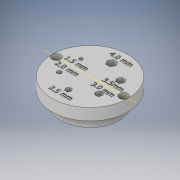
# Autodesk Inventor part: AllenKeyHolder
Saved by Autodesk Inventor 2019.1 (Build 231200000, 200)
## iProperties
Created: 2018-08-31
Part Number: AllenKeyHolder
Material: Generic
Document SubType Name: Modeling
Designer: steele
Density: 1 g/cm^3
Appearance: Default
Author: steele
Autodesk Inventor part; units mm, degrees
(part 1 of 2)
ref_plane "YZ Plane" through (0, 0, 0) normal (1, 0, 0) x (0, 1, 0)
ref_plane "XZ Plane" through (0, 0, 0) normal (0, 1, 0) x (-1, 0, 0)
ref_plane "XY Plane" through (0, 0, 0) normal (0, 0, 1) x (1, 0, 0)
sketch "Sketch1" plane through (0, 0, 0) normal (0, 1, 0) x (-1, 0, 0)
  circle A0 centre (0, 0) radius 20.574
  dimension "d0" = 41.148
  constraints: 1 centre point, 1 coincident
  measures "d0" diameter of A0
extrude "Extrusion1" add sketch "Sketch1" against normal blind 6.35
sketch "Sketch2" plane through (0, -6.35, 0) normal (0, -1, 0) x (1, 0, 0)
  circle A0 centre (0, 0) radius 15.875
  dimension "d3" = 31.75
  constraints: 1 centre point, 1 coincident
  measures "d3" diameter of A0
extrude "Extrusion2" add sketch "Sketch2" along normal blind 6.35
sketch "Sketch4" plane through (0, 0, 0) normal (0, 1, 0) x (1, 0, 0)
  circle A0 centre (0, 0) radius 20.574 projected
  point P0 (18.2245, 0)
  point P1 (-18.2245, 0)
  dimension "d9" = 18.2245
  dimension "d10" = 18.2245
  measures "d9" distance of point (18.224, 0) A0.centre
  measures "d10" distance of point (0, 0) point (-18.224, 0)
hole "Hole1" at (18.2245, 0, 0) at (-18.2245, 0, 0) direction (0, -1, 0) diameter 3.2766 end through all counterbore diameter 4.6482 counterbore depth 2.8448 clearance for "Socket Head Cap Screw" size "#4" standard "Ansi Unified Screw Threads"
sketch "Sketch5" plane through (0, 0, 0) normal (0, 1, 0) x (1, 0, 0)
  circle A0 centre (0, 0) radius 12.065 construction
  line L0 (2.055, 12.0593) -> (0.8425, 9.9593)
  line L1 (0.8425, 9.9593) -> (-1.5823, 9.9593)
  line L2 (-1.5823, 9.9593) -> (-2.7948, 12.0593)
  line L3 (-2.7948, 12.0593) -> (-1.5823, 14.1593)
  line L4 (-1.5823, 14.1593) -> (0.8425, 14.1593)
  line L5 (0.8425, 14.1593) -> (2.055, 12.0593)
  line L6 (12.3949, 6.35) -> (11.3268, 4.5)
  line L7 (11.3268, 4.5) -> (9.1906, 4.5)
  line L8 (9.1906, 4.5) -> (8.1225, 6.35)
  line L9 (8.1225, 6.35) -> (9.1906, 8.2)
  line L10 (9.1906, 8.2) -> (11.3268, 8.2)
  line L11 (11.3268, 8.2) -> (12.3949, 6.35)
  line L12 (-28.8036, 0) -> (28.8036, 0) projected
  line L13 (11.5524, -4.1093) -> (12.4762, -5.7093)
  line L14 (12.4762, -5.7093) -> (11.5524, -7.3093)
  line L15 (11.5524, -7.3093) -> (9.7049, -7.3093)
  line L16 (9.7049, -7.3093) -> (8.7811, -5.7093)
  line L17 (8.7811, -5.7093) -> (9.7049, -4.1093)
  line L18 (9.7049, -4.1093) -> (11.5524, -4.1093)
  line L19 (1.1493, -10.7093) -> (1.9287, -12.0593)
  line L20 (1.9287, -12.0593) -> (1.1493, -13.4093)
  line L21 (1.1493, -13.4093) -> (-0.4095, -13.4093)
  line L22 (-0.4095, -13.4093) -> (-1.189, -12.0593)
  line L23 (-1.189, -12.0593) -> (-0.4095, -10.7093)
  line L24 (-0.4095, -10.7093) -> (1.1493, -10.7093)
  line L25 (-8.9886, -6.35) -> (-9.6237, -7.45)
  line L26 (-9.6237, -7.45) -> (-10.8938, -7.45)
  line L27 (-10.8938, -7.45) -> (-11.5289, -6.35)
  line L28 (-11.5289, -6.35) -> (-10.8938, -5.25)
  line L29 (-10.8938, -5.25) -> (-9.6237, -5.25)
  line L30 (-9.6237, -5.25) -> (-8.9886, -6.35)
  line L31 (-9.6471, 5.7093) -> (-10.1379, 4.8593)
  line L32 (-10.1379, 4.8593) -> (-11.1194, 4.8593)
  line L33 (-11.1194, 4.8593) -> (-11.6101, 5.7093)
  line L34 (-11.6101, 5.7093) -> (-11.1194, 6.5593)
  line L35 (-11.1194, 6.5593) -> (-10.1379, 6.5593)
  line L36 (-10.1379, 6.5593) -> (-9.6471, 5.7093)
  point P0 (-0.3699, 12.0593)
  point P1 (-10.6286, 5.7093)
  point P2 (-10.2587, -6.35)
  point P3 (0.3699, -12.0593)
  point P4 (10.6286, -5.7093)
  point P5 (10.2587, 6.35)
  point P6 (-0.3699, 12.0593)
  point P7 (10.2587, 6.35)
  point P8 (10.6286, -5.7093)
  point P9 (0.3699, -12.0593)
  point P10 (-10.2587, -6.35)
  point P11 (-10.6286, 5.7093)
  dimension "d18" = 24.13
  dimension "d21" = 360
  dimension "d23" = 4.2
  dimension "d24" = 3.7
  dimension "d25" = 3.2
  dimension "d26" = 2.7
  dimension "d27" = 2.2
  dimension "d28" = 1.7
  constraints: 72 end point, 7 coincident, 5 parallel, 88 other
  measures "d23" distance between parallel lines of L1 L4
  measures "d24" distance between parallel lines of L7 L10
  measures "d25" distance between parallel lines of L15 L18
  measures "d26" distance between parallel lines of L21 L24
  measures "d27" distance between parallel lines of L26 L29
  measures "d28" distance between parallel lines of L32 L35
extrude "Extrusion4" cut sketch "Sketch5" against normal through all
sketch "Sketch6" plane through (0, 0, 0) normal (0, 1, 0) x (1, 0, 0)
  line L0 (-12.7271, 15.24) -> (13.8214, 15.24) construction
  circle A0 centre (0, 0) radius 20.574 construction
  line L1 (-11.7818, -16.8665) -> (11.7818, -16.8665) construction
  line L2 (-20.5348, 1.27) -> (20.5348, 1.27) construction
  line L3 (-20.2181, -3.81) -> (20.2181, -3.81) construction
  line L4 (-3.5469, 16.1127) -> (-3.8495, 16.1127)
  line L5 (-3.8495, 16.1127) -> (-3.8495, 15.24)
  line L6 (-3.8495, 15.24) -> (-4.1767, 15.24)
  line L7 (-4.1767, 15.24) -> (-4.1767, 16.1127)
  line L8 (-4.1767, 16.1127) -> (-5.2985, 16.1127)
  line L9 (-5.2985, 16.1127) -> (-5.2985, 16.4709)
  line L10 (-5.2985, 16.4709) -> (-4.1623, 17.78)
  line L11 (-4.1623, 17.78) -> (-3.8495, 17.78)
  line L12 (-3.8495, 17.78) -> (-3.8495, 16.3865)
  line L13 (-3.8495, 16.3865) -> (-3.5469, 16.3865)
  line L14 (-3.5469, 16.3865) -> (-3.5469, 16.1127)
  line L15 (-4.1767, 16.3865) -> (-4.1767, 17.3786)
  line L16 (-4.1767, 17.3786) -> (-5.031, 16.3865)
  line L17 (-5.031, 16.3865) -> (-4.1767, 16.3865)
  line L18 (-2.7297, 15.24) -> (-3.1373, 15.24)
  line L19 (-3.1373, 15.24) -> (-3.1373, 15.7258)
  line L20 (-3.1373, 15.7258) -> (-2.7297, 15.7258)
  line L21 (-2.7297, 15.7258) -> (-2.7297, 15.24)
  spline S0 degree 2 poles (-0.6364, 16.51) (-0.6364, 15.8266) (-1.0337, 15.1865) (-1.4474, 15.1865) knots 0 0 0 1 2 2 2
  spline S1 degree 2 poles (-1.4474, 15.1865) (-1.8673, 15.1865) (-2.2604, 15.839) (-2.2604, 16.5079) knots 0 0 0 1 2 2 2
  spline S2 degree 2 poles (-2.2604, 16.5079) (-2.2604, 17.1954) (-1.8632, 17.8315) (-1.4474, 17.8315) knots 0 0 0 1 2 2 2
  spline S3 degree 2 poles (-1.4474, 17.8315) (-1.0295, 17.8315) (-0.6364, 17.1728) (-0.6364, 16.51) knots 0 0 0 1 2 2 2
  spline S4 degree 2 poles (-1.0728, 15.7361) (-1.0234, 15.8616) (-0.9822, 16.2486) (-0.9822, 16.51) knots 0 0 0 1 2 2 2
  spline S5 degree 2 poles (-0.9822, 16.51) (-0.9822, 16.7714) (-1.0234, 17.1563) (-1.0748, 17.286) knots 0 0 0 1 2 2 2
  spline S6 degree 2 poles (-1.0748, 17.286) (-1.1263, 17.4157) (-1.3054, 17.5495) (-1.4474, 17.5495) knots 0 0 0 1 2 2 2
  spline S7 degree 2 poles (-1.4474, 17.5495) (-1.5894, 17.5495) (-1.7726, 17.4157) (-1.8261, 17.2819) knots 0 0 0 1 2 2 2
  spline S8 degree 2 poles (-1.8261, 17.2819) (-1.8776, 17.1522) (-1.9146, 16.757) (-1.9146, 16.5079) knots 0 0 0 1 2 2 2
  spline S9 degree 2 poles (-1.9146, 16.5079) (-1.9146, 16.2404) (-1.8817, 15.8822) (-1.8282, 15.7422) knots 0 0 0 1 2 2 2
  spline S10 degree 2 poles (-1.8282, 15.7422) (-1.7788, 15.6105) (-1.5956, 15.4685) (-1.4474, 15.4685) knots 0 0 0 1 2 2 2
  spline S11 degree 2 poles (-1.4474, 15.4685) (-1.3074, 15.4685) (-1.1242, 15.6023) (-1.0728, 15.7361) knots 0 0 0 1 2 2 2
  line L22 (2.9884, 15.24) -> (2.9884, 16.3433)
  spline S12 degree 2 poles (2.9884, 16.3433) (2.9884, 16.475) (2.9678, 16.6994) (2.9348, 16.7611) knots 0 0 0 1 2 2 2
  spline S13 degree 2 poles (2.9348, 16.7611) (2.9019, 16.829) (2.7763, 16.8949) (2.6673, 16.8949) knots 0 0 0 1 2 2 2
  spline S14 degree 2 poles (2.6673, 16.8949) (2.5685, 16.8949) (2.342, 16.7735) (2.2227, 16.6582) knots 0 0 0 1 2 2 2
  spline S15 degree 2 poles (2.2227, 16.6582) (2.2247, 16.6294) (2.2288, 16.5491) (2.2288, 16.4956) knots 0 0 0 1 2 2 2
  line L23 (2.2288, 16.4956) -> (2.2288, 15.24)
  line L24 (2.2288, 15.24) -> (1.9077, 15.24)
  line L25 (1.9077, 15.24) -> (1.9077, 16.3433)
  spline S16 degree 2 poles (1.9077, 16.3433) (1.9077, 16.475) (1.8871, 16.6994) (1.8542, 16.7611) knots 0 0 0 1 2 2 2
  spline S17 degree 2 poles (1.8542, 16.7611) (1.8213, 16.829) (1.6957, 16.8949) (1.5866, 16.8949) knots 0 0 0 1 2 2 2
  spline S18 degree 2 poles (1.5866, 16.8949) (1.4837, 16.8949) (1.2552, 16.7652) (1.1482, 16.6644) knots 0 0 0 1 2 2 2
  line L26 (1.1482, 16.6644) -> (1.1482, 15.24)
  line L27 (1.1482, 15.24) -> (0.8271, 15.24)
  line L28 (0.8271, 15.24) -> (0.8271, 17.146)
  line L29 (0.8271, 17.146) -> (1.1482, 17.146)
  line L30 (1.1482, 17.146) -> (1.1482, 16.9361)
  spline S19 degree 2 poles (1.1482, 16.9361) (1.2738, 17.0616) (1.5208, 17.1995) (1.669, 17.1995) knots 0 0 0 1 2 2 2
  spline S20 degree 2 poles (1.669, 17.1995) (1.8377, 17.1995) (2.0992, 17.0452) (2.1671, 16.8702) knots 0 0 0 1 2 2 2
  spline S21 degree 2 poles (2.1671, 16.8702) (2.3132, 17.0328) (2.589, 17.1995) (2.7496, 17.1995) knots 0 0 0 1 2 2 2
  spline S22 degree 2 poles (2.7496, 17.1995) (2.8731, 17.1995) (3.0748, 17.1234) (3.1489, 17.0369) knots 0 0 0 1 2 2 2
  spline S23 degree 2 poles (3.1489, 17.0369) (3.2251, 16.9505) (3.3095, 16.6911) (3.3095, 16.4956) knots 0 0 0 1 2 2 2
  line L31 (3.3095, 16.4956) -> (3.3095, 15.24)
  line L32 (3.3095, 15.24) -> (2.9884, 15.24)
  line L33 (5.9215, 15.24) -> (5.9215, 16.3433)
  spline S24 degree 2 poles (5.9215, 16.3433) (5.9215, 16.475) (5.9009, 16.6994) (5.868, 16.7611) knots 0 0 0 1 2 2 2
  spline S25 degree 2 poles (5.868, 16.7611) (5.8351, 16.829) (5.7095, 16.8949) (5.6004, 16.8949) knots 0 0 0 1 2 2 2
  spline S26 degree 2 poles (5.6004, 16.8949) (5.5016, 16.8949) (5.2752, 16.7735) (5.1558, 16.6582) knots 0 0 0 1 2 2 2
  spline S27 degree 2 poles (5.1558, 16.6582) (5.1579, 16.6294) (5.162, 16.5491) (5.162, 16.4956) knots 0 0 0 1 2 2 2
  line L34 (5.162, 16.4956) -> (5.162, 15.24)
  line L35 (5.162, 15.24) -> (4.8409, 15.24)
  line L36 (4.8409, 15.24) -> (4.8409, 16.3433)
  spline S28 degree 2 poles (4.8409, 16.3433) (4.8409, 16.475) (4.8203, 16.6994) (4.7874, 16.7611) knots 0 0 0 1 2 2 2
  spline S29 degree 2 poles (4.7874, 16.7611) (4.7544, 16.829) (4.6289, 16.8949) (4.5198, 16.8949) knots 0 0 0 1 2 2 2
  spline S30 degree 2 poles (4.5198, 16.8949) (4.4168, 16.8949) (4.1884, 16.7652) (4.0813, 16.6644) knots 0 0 0 1 2 2 2
  line L37 (4.0813, 16.6644) -> (4.0813, 15.24)
  line L38 (4.0813, 15.24) -> (3.7602, 15.24)
  line L39 (3.7602, 15.24) -> (3.7602, 17.146)
  line L40 (3.7602, 17.146) -> (4.0813, 17.146)
  line L41 (4.0813, 17.146) -> (4.0813, 16.9361)
  spline S31 degree 2 poles (4.0813, 16.9361) (4.2069, 17.0616) (4.4539, 17.1995) (4.6021, 17.1995) knots 0 0 0 1 2 2 2
  spline S32 degree 2 poles (4.6021, 17.1995) (4.7709, 17.1995) (5.0323, 17.0452) (5.1002, 16.8702) knots 0 0 0 1 2 2 2
  spline S33 degree 2 poles (5.1002, 16.8702) (5.2464, 17.0328) (5.5222, 17.1995) (5.6827, 17.1995) knots 0 0 0 1 2 2 2
  spline S34 degree 2 poles (5.6827, 17.1995) (5.8062, 17.1995) (6.008, 17.1234) (6.0821, 17.0369) knots 0 0 0 1 2 2 2
  spline S35 degree 2 poles (6.0821, 17.0369) (6.1582, 16.9505) (6.2426, 16.6911) (6.2426, 16.4956) knots 0 0 0 1 2 2 2
  line L42 (6.2426, 16.4956) -> (6.2426, 15.24)
  line L43 (6.2426, 15.24) -> (5.9215, 15.24)
  line L44 (-14.0215, 1.27) -> (-15.2606, 1.27)
  line L45 (-15.2606, 1.27) -> (-15.2606, 1.5294)
  line L46 (-15.2606, 1.5294) -> (-14.7995, 1.5294)
  line L47 (-14.7995, 1.5294) -> (-14.7995, 3.2316)
  line L48 (-14.7995, 3.2316) -> (-15.2606, 3.2316)
  line L49 (-15.2606, 3.2316) -> (-15.2606, 3.4642)
  spline S36 degree 2 poles (-15.2606, 3.4642) (-14.9992, 3.4642) (-14.7522, 3.6124) (-14.7357, 3.8182) knots 0 0 0 1 2 2 2
  line L50 (-14.7357, 3.8182) -> (-14.4722, 3.8182)
  line L51 (-14.4722, 3.8182) -> (-14.4722, 1.5294)
  line L52 (-14.4722, 1.5294) -> (-14.0215, 1.5294)
  line L53 (-14.0215, 1.5294) -> (-14.0215, 1.27)
  line L54 (-13.0088, 1.27) -> (-13.4163, 1.27)
  line L55 (-13.4163, 1.27) -> (-13.4163, 1.7558)
  line L56 (-13.4163, 1.7558) -> (-13.0088, 1.7558)
  line L57 (-13.0088, 1.7558) -> (-13.0088, 1.27)
  spline S37 degree 2 poles (-10.9566, 2.0769) (-10.9566, 1.8937) (-11.0739, 1.5808) (-11.1809, 1.4655) knots 0 0 0 1 2 2 2
  spline S38 degree 2 poles (-11.1809, 1.4655) (-11.288, 1.3503) (-11.607, 1.2165) (-11.8046, 1.2165) knots 0 0 0 1 2 2 2
  spline S39 degree 2 poles (-11.8046, 1.2165) (-11.9858, 1.2165) (-12.3398, 1.2968) (-12.4695, 1.3606) knots 0 0 0 1 2 2 2
  line L58 (-12.4695, 1.3606) -> (-12.4695, 1.7208)
  line L59 (-12.4695, 1.7208) -> (-12.4448, 1.7208)
  spline S40 degree 2 poles (-12.4448, 1.7208) (-12.4057, 1.692) (-12.2595, 1.6179) (-12.171, 1.5849) knots 0 0 0 1 2 2 2
  spline S41 degree 2 poles (-12.171, 1.5849) (-12.0701, 1.5499) (-11.9034, 1.5108) (-11.7984, 1.5108) knots 0 0 0 1 2 2 2
  spline S42 degree 2 poles (-11.7984, 1.5108) (-11.6955, 1.5108) (-11.502, 1.5849) (-11.4321, 1.6652) knots 0 0 0 1 2 2 2
  spline S43 degree 2 poles (-11.4321, 1.6652) (-11.3682, 1.7414) (-11.3024, 1.9431) (-11.3024, 2.0789) knots 0 0 0 1 2 2 2
  spline S44 degree 2 poles (-11.3024, 2.0789) (-11.3024, 2.2148) (-11.3765, 2.3877) (-11.4465, 2.4453) knots 0 0 0 1 2 2 2
  spline S45 degree 2 poles (-11.4465, 2.4453) (-11.5185, 2.5091) (-11.7326, 2.5626) (-11.8623, 2.5626) knots 0 0 0 1 2 2 2
  spline S46 degree 2 poles (-11.8623, 2.5626) (-12.0022, 2.5626) (-12.2801, 2.5194) (-12.3645, 2.5009) knots 0 0 0 1 2 2 2
  line L60 (-12.3645, 2.5009) -> (-12.3645, 3.81)
  line L61 (-12.3645, 3.81) -> (-10.971, 3.81)
  line L62 (-10.971, 3.81) -> (-10.971, 3.5115)
  line L63 (-10.971, 3.5115) -> (-12.0372, 3.5115)
  line L64 (-12.0372, 3.5115) -> (-12.0372, 2.8343)
  spline S47 degree 2 poles (-12.0372, 2.8343) (-11.9755, 2.8426) (-11.8561, 2.8488) (-11.8067, 2.8488) knots 0 0 0 1 2 2 2
  spline S48 degree 2 poles (-11.8067, 2.8488) (-11.6111, 2.8488) (-11.3415, 2.7849) (-11.218, 2.6903) knots 0 0 0 1 2 2 2
  spline S49 degree 2 poles (-11.218, 2.6903) (-11.0924, 2.5956) (-10.9566, 2.3074) (-10.9566, 2.0769) knots 0 0 0 1 2 2 2
  line L65 (-7.2907, 1.27) -> (-7.2907, 2.3733)
  spline S50 degree 2 poles (-7.2907, 2.3733) (-7.2907, 2.505) (-7.3112, 2.7294) (-7.3442, 2.7911) knots 0 0 0 1 2 2 2
  spline S51 degree 2 poles (-7.3442, 2.7911) (-7.3771, 2.859) (-7.5027, 2.9249) (-7.6118, 2.9249) knots 0 0 0 1 2 2 2
  spline S52 degree 2 poles (-7.6118, 2.9249) (-7.7106, 2.9249) (-7.937, 2.8035) (-8.0564, 2.6882) knots 0 0 0 1 2 2 2
  spline S53 degree 2 poles (-8.0564, 2.6882) (-8.0543, 2.6594) (-8.0502, 2.5791) (-8.0502, 2.5256) knots 0 0 0 1 2 2 2
  line L66 (-8.0502, 2.5256) -> (-8.0502, 1.27)
  line L67 (-8.0502, 1.27) -> (-8.3713, 1.27)
  line L68 (-8.3713, 1.27) -> (-8.3713, 2.3733)
  spline S54 degree 2 poles (-8.3713, 2.3733) (-8.3713, 2.505) (-8.3919, 2.7294) (-8.4248, 2.7911) knots 0 0 0 1 2 2 2
  spline S55 degree 2 poles (-8.4248, 2.7911) (-8.4577, 2.859) (-8.5833, 2.9249) (-8.6924, 2.9249) knots 0 0 0 1 2 2 2
  spline S56 degree 2 poles (-8.6924, 2.9249) (-8.7953, 2.9249) (-9.0238, 2.7952) (-9.1308, 2.6944) knots 0 0 0 1 2 2 2
  line L69 (-9.1308, 2.6944) -> (-9.1308, 1.27)
  line L70 (-9.1308, 1.27) -> (-9.4519, 1.27)
  line L71 (-9.4519, 1.27) -> (-9.4519, 3.176)
  line L72 (-9.4519, 3.176) -> (-9.1308, 3.176)
  line L73 (-9.1308, 3.176) -> (-9.1308, 2.9661)
  spline S57 degree 2 poles (-9.1308, 2.9661) (-9.0053, 3.0916) (-8.7583, 3.2295) (-8.6101, 3.2295) knots 0 0 0 1 2 2 2
  spline S58 degree 2 poles (-8.6101, 3.2295) (-8.4413, 3.2295) (-8.1799, 3.0752) (-8.1119, 2.9002) knots 0 0 0 1 2 2 2
  spline S59 degree 2 poles (-8.1119, 2.9002) (-7.9658, 3.0628) (-7.69, 3.2295) (-7.5294, 3.2295) knots 0 0 0 1 2 2 2
  spline S60 degree 2 poles (-7.5294, 3.2295) (-7.4059, 3.2295) (-7.2042, 3.1534) (-7.1301, 3.0669) knots 0 0 0 1 2 2 2
  spline S61 degree 2 poles (-7.1301, 3.0669) (-7.054, 2.9805) (-6.9696, 2.7211) (-6.9696, 2.5256) knots 0 0 0 1 2 2 2
  line L74 (-6.9696, 2.5256) -> (-6.9696, 1.27)
  line L75 (-6.9696, 1.27) -> (-7.2907, 1.27)
  line L76 (-4.3575, 1.27) -> (-4.3575, 2.3733)
  spline S62 degree 2 poles (-4.3575, 2.3733) (-4.3575, 2.505) (-4.3781, 2.7294) (-4.411, 2.7911) knots 0 0 0 1 2 2 2
  spline S63 degree 2 poles (-4.411, 2.7911) (-4.444, 2.859) (-4.5695, 2.9249) (-4.6786, 2.9249) knots 0 0 0 1 2 2 2
  spline S64 degree 2 poles (-4.6786, 2.9249) (-4.7774, 2.9249) (-5.0038, 2.8035) (-5.1232, 2.6882) knots 0 0 0 1 2 2 2
  spline S65 degree 2 poles (-5.1232, 2.6882) (-5.1212, 2.6594) (-5.1171, 2.5791) (-5.1171, 2.5256) knots 0 0 0 1 2 2 2
  line L77 (-5.1171, 2.5256) -> (-5.1171, 1.27)
  line L78 (-5.1171, 1.27) -> (-5.4382, 1.27)
  line L79 (-5.4382, 1.27) -> (-5.4382, 2.3733)
  spline S66 degree 2 poles (-5.4382, 2.3733) (-5.4382, 2.505) (-5.4587, 2.7294) (-5.4917, 2.7911) knots 0 0 0 1 2 2 2
  spline S67 degree 2 poles (-5.4917, 2.7911) (-5.5246, 2.859) (-5.6502, 2.9249) (-5.7593, 2.9249) knots 0 0 0 1 2 2 2
  spline S68 degree 2 poles (-5.7593, 2.9249) (-5.8622, 2.9249) (-6.0906, 2.7952) (-6.1977, 2.6944) knots 0 0 0 1 2 2 2
  line L80 (-6.1977, 2.6944) -> (-6.1977, 1.27)
  line L81 (-6.1977, 1.27) -> (-6.5188, 1.27)
  line L82 (-6.5188, 1.27) -> (-6.5188, 3.176)
  line L83 (-6.5188, 3.176) -> (-6.1977, 3.176)
  line L84 (-6.1977, 3.176) -> (-6.1977, 2.9661)
  spline S69 degree 2 poles (-6.1977, 2.9661) (-6.0721, 3.0916) (-5.8251, 3.2295) (-5.6769, 3.2295) knots 0 0 0 1 2 2 2
  spline S70 degree 2 poles (-5.6769, 3.2295) (-5.5081, 3.2295) (-5.2467, 3.0752) (-5.1788, 2.9002) knots 0 0 0 1 2 2 2
  spline S71 degree 2 poles (-5.1788, 2.9002) (-5.0327, 3.0628) (-4.7568, 3.2295) (-4.5963, 3.2295) knots 0 0 0 1 2 2 2
  spline S72 degree 2 poles (-4.5963, 3.2295) (-4.4728, 3.2295) (-4.2711, 3.1534) (-4.197, 3.0669) knots 0 0 0 1 2 2 2
  spline S73 degree 2 poles (-4.197, 3.0669) (-4.1208, 2.9805) (-4.0364, 2.7211) (-4.0364, 2.5256) knots 0 0 0 1 2 2 2
  line L85 (-4.0364, 2.5256) -> (-4.0364, 1.27)
  line L86 (-4.0364, 1.27) -> (-4.3575, 1.27)
  spline S74 degree 2 poles (5.7798, 3.5692) (5.6872, 3.5692) (5.504, 3.5239) (5.4155, 3.4889) knots 0 0 0 1 2 2 2
  spline S75 degree 2 poles (5.4155, 3.4889) (5.3332, 3.4539) (5.2117, 3.3798) (5.1644, 3.3469) knots 0 0 0 1 2 2 2
  line L87 (5.1644, 3.3469) -> (5.1438, 3.3469)
  line L88 (5.1438, 3.3469) -> (5.1438, 3.7071)
  spline S76 degree 2 poles (5.1438, 3.7071) (5.255, 3.7668) (5.6358, 3.8635) (5.8066, 3.8635) knots 0 0 0 1 2 2 2
  spline S77 degree 2 poles (5.8066, 3.8635) (5.9795, 3.8635) (6.2368, 3.7935) (6.3418, 3.7194) knots 0 0 0 1 2 2 2
  spline S78 degree 2 poles (6.3418, 3.7194) (6.4529, 3.6392) (6.5682, 3.4066) (6.5682, 3.2501) knots 0 0 0 1 2 2 2
  spline S79 degree 2 poles (6.5682, 3.2501) (6.5682, 3.0402) (6.2924, 2.7232) (6.0989, 2.682) knots 0 0 0 1 2 2 2
  line L89 (6.0989, 2.682) -> (6.0989, 2.6573)
  spline S80 degree 2 poles (6.0989, 2.6573) (6.1792, 2.6409) (6.3624, 2.5668) (6.4406, 2.4927) knots 0 0 0 1 2 2 2
  spline S81 degree 2 poles (6.4406, 2.4927) (6.5188, 2.4206) (6.6176, 2.1901) (6.6176, 2.0234) knots 0 0 0 1 2 2 2
  spline S82 degree 2 poles (6.6176, 2.0234) (6.6176, 1.8525) (6.5003, 1.5623) (6.3932, 1.4511) knots 0 0 0 1 2 2 2
  spline S83 degree 2 poles (6.3932, 1.4511) (6.2821, 1.3359) (5.9671, 1.2165) (5.7675, 1.2165) knots 0 0 0 1 2 2 2
  spline S84 degree 2 poles (5.7675, 1.2165) (5.5761, 1.2165) (5.2014, 1.3091) (5.0738, 1.3729) knots 0 0 0 1 2 2 2
  line L90 (5.0738, 1.3729) -> (5.0738, 1.7331)
  line L91 (5.0738, 1.7331) -> (5.0985, 1.7331)
  spline S85 degree 2 poles (5.0985, 1.7331) (5.2056, 1.6549) (5.5678, 1.5108) (5.7469, 1.5108) knots 0 0 0 1 2 2 2
  spline S86 degree 2 poles (5.7469, 1.5108) (5.8519, 1.5108) (6.0618, 1.5767) (6.1318, 1.6529) knots 0 0 0 1 2 2 2
  spline S87 degree 2 poles (6.1318, 1.6529) (6.1997, 1.729) (6.2718, 1.9101) (6.2718, 2.0481) knots 0 0 0 1 2 2 2
  spline S88 degree 2 poles (6.2718, 2.0481) (6.2718, 2.186) (6.1915, 2.365) (6.1195, 2.4165) knots 0 0 0 1 2 2 2
  spline S89 degree 2 poles (6.1195, 2.4165) (6.0474, 2.468) (5.8519, 2.5071) (5.7366, 2.5071) knots 0 0 0 1 2 2 2
  line L92 (5.7366, 2.5071) -> (5.5925, 2.5071)
  line L93 (5.5925, 2.5071) -> (5.5925, 2.7891)
  line L94 (5.5925, 2.7891) -> (5.7057, 2.7891)
  spline S90 degree 2 poles (5.7057, 2.7891) (5.9342, 2.7891) (6.2224, 3.0072) (6.2224, 3.2151) knots 0 0 0 1 2 2 2
  spline S91 degree 2 poles (6.2224, 3.2151) (6.2224, 3.3119) (6.1483, 3.4498) (6.0886, 3.491) knots 0 0 0 1 2 2 2
  spline S92 degree 2 poles (6.0886, 3.491) (6.0248, 3.5342) (5.8683, 3.5692) (5.7798, 3.5692) knots 0 0 0 1 2 2 2
  line L95 (7.5459, 1.27) -> (7.1383, 1.27)
  line L96 (7.1383, 1.27) -> (7.1383, 1.7558)
  line L97 (7.1383, 1.7558) -> (7.5459, 1.7558)
  line L98 (7.5459, 1.7558) -> (7.5459, 1.27)
  spline S93 degree 2 poles (9.5981, 2.0769) (9.5981, 1.8937) (9.4807, 1.5808) (9.3737, 1.4655) knots 0 0 0 1 2 2 2
  spline S94 degree 2 poles (9.3737, 1.4655) (9.2667, 1.3503) (8.9476, 1.2165) (8.75, 1.2165) knots 0 0 0 1 2 2 2
  spline S95 degree 2 poles (8.75, 1.2165) (8.5689, 1.2165) (8.2149, 1.2968) (8.0852, 1.3606) knots 0 0 0 1 2 2 2
  line L99 (8.0852, 1.3606) -> (8.0852, 1.7208)
  line L100 (8.0852, 1.7208) -> (8.1099, 1.7208)
  spline S96 degree 2 poles (8.1099, 1.7208) (8.149, 1.692) (8.2951, 1.6179) (8.3836, 1.5849) knots 0 0 0 1 2 2 2
  spline S97 degree 2 poles (8.3836, 1.5849) (8.4845, 1.5499) (8.6512, 1.5108) (8.7562, 1.5108) knots 0 0 0 1 2 2 2
  spline S98 degree 2 poles (8.7562, 1.5108) (8.8591, 1.5108) (9.0526, 1.5849) (9.1226, 1.6652) knots 0 0 0 1 2 2 2
  spline S99 degree 2 poles (9.1226, 1.6652) (9.1864, 1.7414) (9.2523, 1.9431) (9.2523, 2.0789) knots 0 0 0 1 2 2 2
  spline S100 degree 2 poles (9.2523, 2.0789) (9.2523, 2.2148) (9.1782, 2.3877) (9.1082, 2.4453) knots 0 0 0 1 2 2 2
  spline S101 degree 2 poles (9.1082, 2.4453) (9.0361, 2.5091) (8.8221, 2.5626) (8.6924, 2.5626) knots 0 0 0 1 2 2 2
  spline S102 degree 2 poles (8.6924, 2.5626) (8.5524, 2.5626) (8.2746, 2.5194) (8.1902, 2.5009) knots 0 0 0 1 2 2 2
  line L101 (8.1902, 2.5009) -> (8.1902, 3.81)
  line L102 (8.1902, 3.81) -> (9.5837, 3.81)
  line L103 (9.5837, 3.81) -> (9.5837, 3.5115)
  line L104 (9.5837, 3.5115) -> (8.5174, 3.5115)
  line L105 (8.5174, 3.5115) -> (8.5174, 2.8343)
  spline S103 degree 2 poles (8.5174, 2.8343) (8.5792, 2.8426) (8.6986, 2.8488) (8.748, 2.8488) knots 0 0 0 1 2 2 2
  spline S104 degree 2 poles (8.748, 2.8488) (8.9435, 2.8488) (9.2132, 2.7849) (9.3367, 2.6903) knots 0 0 0 1 2 2 2
  spline S105 degree 2 poles (9.3367, 2.6903) (9.4622, 2.5956) (9.5981, 2.3074) (9.5981, 2.0769) knots 0 0 0 1 2 2 2
  line L106 (12.1731, 1.27) -> (12.1731, 2.3733)
  spline S106 degree 2 poles (12.1731, 2.3733) (12.1731, 2.505) (12.1525, 2.7294) (12.1195, 2.7911) knots 0 0 0 1 2 2 2
  spline S107 degree 2 poles (12.1195, 2.7911) (12.0866, 2.859) (11.9611, 2.9249) (11.852, 2.9249) knots 0 0 0 1 2 2 2
  spline S108 degree 2 poles (11.852, 2.9249) (11.7532, 2.9249) (11.5267, 2.8035) (11.4074, 2.6882) knots 0 0 0 1 2 2 2
  spline S109 degree 2 poles (11.4074, 2.6882) (11.4094, 2.6594) (11.4135, 2.5791) (11.4135, 2.5256) knots 0 0 0 1 2 2 2
  line L107 (11.4135, 2.5256) -> (11.4135, 1.27)
  line L108 (11.4135, 1.27) -> (11.0924, 1.27)
  line L109 (11.0924, 1.27) -> (11.0924, 2.3733)
  spline S110 degree 2 poles (11.0924, 2.3733) (11.0924, 2.505) (11.0718, 2.7294) (11.0389, 2.7911) knots 0 0 0 1 2 2 2
  spline S111 degree 2 poles (11.0389, 2.7911) (11.006, 2.859) (10.8804, 2.9249) (10.7713, 2.9249) knots 0 0 0 1 2 2 2
  spline S112 degree 2 poles (10.7713, 2.9249) (10.6684, 2.9249) (10.4399, 2.7952) (10.3329, 2.6944) knots 0 0 0 1 2 2 2
  line L110 (10.3329, 2.6944) -> (10.3329, 1.27)
  line L111 (10.3329, 1.27) -> (10.0118, 1.27)
  line L112 (10.0118, 1.27) -> (10.0118, 3.176)
  line L113 (10.0118, 3.176) -> (10.3329, 3.176)
  line L114 (10.3329, 3.176) -> (10.3329, 2.9661)
  spline S113 degree 2 poles (10.3329, 2.9661) (10.4585, 3.0916) (10.7055, 3.2295) (10.8537, 3.2295) knots 0 0 0 1 2 2 2
  spline S114 degree 2 poles (10.8537, 3.2295) (11.0224, 3.2295) (11.2839, 3.0752) (11.3518, 2.9002) knots 0 0 0 1 2 2 2
  spline S115 degree 2 poles (11.3518, 2.9002) (11.4979, 3.0628) (11.7737, 3.2295) (11.9343, 3.2295) knots 0 0 0 1 2 2 2
  spline S116 degree 2 poles (11.9343, 3.2295) (12.0578, 3.2295) (12.2595, 3.1534) (12.3336, 3.0669) knots 0 0 0 1 2 2 2
  spline S117 degree 2 poles (12.3336, 3.0669) (12.4098, 2.9805) (12.4942, 2.7211) (12.4942, 2.5256) knots 0 0 0 1 2 2 2
  line L115 (12.4942, 2.5256) -> (12.4942, 1.27)
  line L116 (12.4942, 1.27) -> (12.1731, 1.27)
  line L117 (15.1062, 1.27) -> (15.1062, 2.3733)
  spline S118 degree 2 poles (15.1062, 2.3733) (15.1062, 2.505) (15.0856, 2.7294) (15.0527, 2.7911) knots 0 0 0 1 2 2 2
  spline S119 degree 2 poles (15.0527, 2.7911) (15.0198, 2.859) (14.8942, 2.9249) (14.7851, 2.9249) knots 0 0 0 1 2 2 2
  spline S120 degree 2 poles (14.7851, 2.9249) (14.6863, 2.9249) (14.4599, 2.8035) (14.3405, 2.6882) knots 0 0 0 1 2 2 2
  spline S121 degree 2 poles (14.3405, 2.6882) (14.3426, 2.6594) (14.3467, 2.5791) (14.3467, 2.5256) knots 0 0 0 1 2 2 2
  line L118 (14.3467, 2.5256) -> (14.3467, 1.27)
  line L119 (14.3467, 1.27) -> (14.0256, 1.27)
  line L120 (14.0256, 1.27) -> (14.0256, 2.3733)
  spline S122 degree 2 poles (14.0256, 2.3733) (14.0256, 2.505) (14.005, 2.7294) (13.9721, 2.7911) knots 0 0 0 1 2 2 2
  spline S123 degree 2 poles (13.9721, 2.7911) (13.9391, 2.859) (13.8136, 2.9249) (13.7045, 2.9249) knots 0 0 0 1 2 2 2
  spline S124 degree 2 poles (13.7045, 2.9249) (13.6016, 2.9249) (13.3731, 2.7952) (13.266, 2.6944) knots 0 0 0 1 2 2 2
  line L121 (13.266, 2.6944) -> (13.266, 1.27)
  line L122 (13.266, 1.27) -> (12.9449, 1.27)
  line L123 (12.9449, 1.27) -> (12.9449, 3.176)
  line L124 (12.9449, 3.176) -> (13.266, 3.176)
  line L125 (13.266, 3.176) -> (13.266, 2.9661)
  spline S125 degree 2 poles (13.266, 2.9661) (13.3916, 3.0916) (13.6386, 3.2295) (13.7868, 3.2295) knots 0 0 0 1 2 2 2
  spline S126 degree 2 poles (13.7868, 3.2295) (13.9556, 3.2295) (14.217, 3.0752) (14.2849, 2.9002) knots 0 0 0 1 2 2 2
  spline S127 degree 2 poles (14.2849, 2.9002) (14.4311, 3.0628) (14.7069, 3.2295) (14.8674, 3.2295) knots 0 0 0 1 2 2 2
  spline S128 degree 2 poles (14.8674, 3.2295) (14.9909, 3.2295) (15.1927, 3.1534) (15.2668, 3.0669) knots 0 0 0 1 2 2 2
  spline S129 degree 2 poles (15.2668, 3.0669) (15.3429, 2.9805) (15.4273, 2.7211) (15.4273, 2.5256) knots 0 0 0 1 2 2 2
  line L126 (15.4273, 2.5256) -> (15.4273, 1.27)
  line L127 (15.4273, 1.27) -> (15.1062, 1.27)
  line L128 (-13.8938, -3.81) -> (-15.4602, -3.81)
  line L129 (-15.4602, -3.81) -> (-15.4602, -3.4498)
  spline S130 degree 2 poles (-15.4602, -3.4498) (-15.2915, -3.2913) (-14.9909, -2.997) (-14.8469, -2.8385) knots 0 0 0 1 2 2 2
  spline S131 degree 2 poles (-14.8469, -2.8385) (-14.5566, -2.5194) (-14.3446, -2.1366) (-14.3446, -1.9328) knots 0 0 0 1 2 2 2
  spline S132 degree 2 poles (-14.3446, -1.9328) (-14.3446, -1.8258) (-14.4105, -1.6652) (-14.4702, -1.6137) knots 0 0 0 1 2 2 2
  spline S133 degree 2 poles (-14.4702, -1.6137) (-14.5299, -1.5623) (-14.6863, -1.5108) (-14.781, -1.5108) knots 0 0 0 1 2 2 2
  spline S134 degree 2 poles (-14.781, -1.5108) (-14.8716, -1.5108) (-15.0568, -1.5561) (-15.1412, -1.5911) knots 0 0 0 1 2 2 2
  spline S135 degree 2 poles (-15.1412, -1.5911) (-15.2132, -1.6199) (-15.347, -1.7023) (-15.3882, -1.7311) knots 0 0 0 1 2 2 2
  line L130 (-15.3882, -1.7311) -> (-15.4067, -1.7311)
  line L131 (-15.4067, -1.7311) -> (-15.4067, -1.3688)
  spline S136 degree 2 poles (-15.4067, -1.3688) (-15.3018, -1.3173) (-14.9251, -1.2165) (-14.7563, -1.2165) knots 0 0 0 1 2 2 2
  spline S137 degree 2 poles (-14.7563, -1.2165) (-14.4002, -1.2165) (-13.9988, -1.5932) (-13.9988, -1.9143) knots 0 0 0 1 2 2 2
  spline S138 degree 2 poles (-13.9988, -1.9143) (-13.9988, -2.0645) (-14.0688, -2.3156) (-14.1306, -2.4227) knots 0 0 0 1 2 2 2
  spline S139 degree 2 poles (-14.1306, -2.4227) (-14.1923, -2.5338) (-14.3714, -2.752) (-14.4702, -2.857) knots 0 0 0 1 2 2 2
  spline S140 degree 2 poles (-14.4702, -2.857) (-14.6307, -3.0319) (-15.0239, -3.4066) (-15.1412, -3.5157) knots 0 0 0 1 2 2 2
  line L132 (-15.1412, -3.5157) -> (-13.8938, -3.5157)
  line L133 (-13.8938, -3.5157) -> (-13.8938, -3.81)
  line L134 (-13.0088, -3.81) -> (-13.4163, -3.81)
  line L135 (-13.4163, -3.81) -> (-13.4163, -3.3242)
  line L136 (-13.4163, -3.3242) -> (-13.0088, -3.3242)
  line L137 (-13.0088, -3.3242) -> (-13.0088, -3.81)
  spline S141 degree 2 poles (-10.9154, -2.54) (-10.9154, -3.2234) (-11.3127, -3.8635) (-11.7264, -3.8635) knots 0 0 0 1 2 2 2
  spline S142 degree 2 poles (-11.7264, -3.8635) (-12.1463, -3.8635) (-12.5394, -3.211) (-12.5394, -2.5421) knots 0 0 0 1 2 2 2
  spline S143 degree 2 poles (-12.5394, -2.5421) (-12.5394, -1.8546) (-12.1422, -1.2185) (-11.7264, -1.2185) knots 0 0 0 1 2 2 2
  spline S144 degree 2 poles (-11.7264, -1.2185) (-11.3086, -1.2185) (-10.9154, -1.8772) (-10.9154, -2.54) knots 0 0 0 1 2 2 2
  spline S145 degree 2 poles (-11.3518, -3.3139) (-11.3024, -3.1884) (-11.2612, -2.8014) (-11.2612, -2.54) knots 0 0 0 1 2 2 2
  spline S146 degree 2 poles (-11.2612, -2.54) (-11.2612, -2.2786) (-11.3024, -1.8937) (-11.3538, -1.764) knots 0 0 0 1 2 2 2
  spline S147 degree 2 poles (-11.3538, -1.764) (-11.4053, -1.6343) (-11.5844, -1.5005) (-11.7264, -1.5005) knots 0 0 0 1 2 2 2
  spline S148 degree 2 poles (-11.7264, -1.5005) (-11.8684, -1.5005) (-12.0516, -1.6343) (-12.1051, -1.7681) knots 0 0 0 1 2 2 2
  spline S149 degree 2 poles (-12.1051, -1.7681) (-12.1566, -1.8978) (-12.1936, -2.293) (-12.1936, -2.5421) knots 0 0 0 1 2 2 2
  spline S150 degree 2 poles (-12.1936, -2.5421) (-12.1936, -2.8096) (-12.1607, -3.1678) (-12.1072, -3.3078) knots 0 0 0 1 2 2 2
  spline S151 degree 2 poles (-12.1072, -3.3078) (-12.0578, -3.4395) (-11.8746, -3.5815) (-11.7264, -3.5815) knots 0 0 0 1 2 2 2
  spline S152 degree 2 poles (-11.7264, -3.5815) (-11.5864, -3.5815) (-11.4032, -3.4477) (-11.3518, -3.3139) knots 0 0 0 1 2 2 2
  line L138 (-7.2907, -3.81) -> (-7.2907, -2.7067)
  spline S153 degree 2 poles (-7.2907, -2.7067) (-7.2907, -2.575) (-7.3112, -2.3506) (-7.3442, -2.2889) knots 0 0 0 1 2 2 2
  spline S154 degree 2 poles (-7.3442, -2.2889) (-7.3771, -2.221) (-7.5027, -2.1551) (-7.6118, -2.1551) knots 0 0 0 1 2 2 2
  spline S155 degree 2 poles (-7.6118, -2.1551) (-7.7106, -2.1551) (-7.937, -2.2765) (-8.0564, -2.3918) knots 0 0 0 1 2 2 2
  spline S156 degree 2 poles (-8.0564, -2.3918) (-8.0543, -2.4206) (-8.0502, -2.5009) (-8.0502, -2.5544) knots 0 0 0 1 2 2 2
  line L139 (-8.0502, -2.5544) -> (-8.0502, -3.81)
  line L140 (-8.0502, -3.81) -> (-8.3713, -3.81)
  line L141 (-8.3713, -3.81) -> (-8.3713, -2.7067)
  spline S157 degree 2 poles (-8.3713, -2.7067) (-8.3713, -2.575) (-8.3919, -2.3506) (-8.4248, -2.2889) knots 0 0 0 1 2 2 2
  spline S158 degree 2 poles (-8.4248, -2.2889) (-8.4577, -2.221) (-8.5833, -2.1551) (-8.6924, -2.1551) knots 0 0 0 1 2 2 2
  spline S159 degree 2 poles (-8.6924, -2.1551) (-8.7953, -2.1551) (-9.0238, -2.2848) (-9.1308, -2.3856) knots 0 0 0 1 2 2 2
  line L142 (-9.1308, -2.3856) -> (-9.1308, -3.81)
  line L143 (-9.1308, -3.81) -> (-9.4519, -3.81)
  line L144 (-9.4519, -3.81) -> (-9.4519, -1.904)
  line L145 (-9.4519, -1.904) -> (-9.1308, -1.904)
  line L146 (-9.1308, -1.904) -> (-9.1308, -2.1139)
  spline S160 degree 2 poles (-9.1308, -2.1139) (-9.0053, -1.9884) (-8.7583, -1.8505) (-8.6101, -1.8505) knots 0 0 0 1 2 2 2
  spline S161 degree 2 poles (-8.6101, -1.8505) (-8.4413, -1.8505) (-8.1799, -2.0048) (-8.1119, -2.1798) knots 0 0 0 1 2 2 2
  spline S162 degree 2 poles (-8.1119, -2.1798) (-7.9658, -2.0172) (-7.69, -1.8505) (-7.5294, -1.8505) knots 0 0 0 1 2 2 2
  spline S163 degree 2 poles (-7.5294, -1.8505) (-7.4059, -1.8505) (-7.2042, -1.9266) (-7.1301, -2.0131) knots 0 0 0 1 2 2 2
  spline S164 degree 2 poles (-7.1301, -2.0131) (-7.054, -2.0995) (-6.9696, -2.3589) (-6.9696, -2.5544) knots 0 0 0 1 2 2 2
  line L147 (-6.9696, -2.5544) -> (-6.9696, -3.81)
  line L148 (-6.9696, -3.81) -> (-7.2907, -3.81)
  line L149 (-4.3575, -3.81) -> (-4.3575, -2.7067)
  spline S165 degree 2 poles (-4.3575, -2.7067) (-4.3575, -2.575) (-4.3781, -2.3506) (-4.411, -2.2889) knots 0 0 0 1 2 2 2
  spline S166 degree 2 poles (-4.411, -2.2889) (-4.444, -2.221) (-4.5695, -2.1551) (-4.6786, -2.1551) knots 0 0 0 1 2 2 2
  spline S167 degree 2 poles (-4.6786, -2.1551) (-4.7774, -2.1551) (-5.0038, -2.2765) (-5.1232, -2.3918) knots 0 0 0 1 2 2 2
  spline S168 degree 2 poles (-5.1232, -2.3918) (-5.1212, -2.4206) (-5.1171, -2.5009) (-5.1171, -2.5544) knots 0 0 0 1 2 2 2
  line L150 (-5.1171, -2.5544) -> (-5.1171, -3.81)
  line L151 (-5.1171, -3.81) -> (-5.4382, -3.81)
  line L152 (-5.4382, -3.81) -> (-5.4382, -2.7067)
  spline S169 degree 2 poles (-5.4382, -2.7067) (-5.4382, -2.575) (-5.4587, -2.3506) (-5.4917, -2.2889) knots 0 0 0 1 2 2 2
  spline S170 degree 2 poles (-5.4917, -2.2889) (-5.5246, -2.221) (-5.6502, -2.1551) (-5.7593, -2.1551) knots 0 0 0 1 2 2 2
  spline S171 degree 2 poles (-5.7593, -2.1551) (-5.8622, -2.1551) (-6.0906, -2.2848) (-6.1977, -2.3856) knots 0 0 0 1 2 2 2
  line L153 (-6.1977, -2.3856) -> (-6.1977, -3.81)
  line L154 (-6.1977, -3.81) -> (-6.5188, -3.81)
  line L155 (-6.5188, -3.81) -> (-6.5188, -1.904)
  line L156 (-6.5188, -1.904) -> (-6.1977, -1.904)
  line L157 (-6.1977, -1.904) -> (-6.1977, -2.1139)
  spline S172 degree 2 poles (-6.1977, -2.1139) (-6.0721, -1.9884) (-5.8251, -1.8505) (-5.6769, -1.8505) knots 0 0 0 1 2 2 2
  spline S173 degree 2 poles (-5.6769, -1.8505) (-5.5081, -1.8505) (-5.2467, -2.0048) (-5.1788, -2.1798) knots 0 0 0 1 2 2 2
  spline S174 degree 2 poles (-5.1788, -2.1798) (-5.0327, -2.0172) (-4.7568, -1.8505) (-4.5963, -1.8505) knots 0 0 0 1 2 2 2
  spline S175 degree 2 poles (-4.5963, -1.8505) (-4.4728, -1.8505) (-4.2711, -1.9266) (-4.197, -2.0131) knots 0 0 0 1 2 2 2
  spline S176 degree 2 poles (-4.197, -2.0131) (-4.1208, -2.0995) (-4.0364, -2.3589) (-4.0364, -2.5544) knots 0 0 0 1 2 2 2
  line L158 (-4.0364, -2.5544) -> (-4.0364, -3.81)
  line L159 (-4.0364, -3.81) -> (-4.3575, -3.81)
  spline S177 degree 2 poles (4.6889, -1.5108) (4.5963, -1.5108) (4.4131, -1.5561) (4.3246, -1.5911) knots 0 0 0 1 2 2 2
  spline S178 degree 2 poles (4.3246, -1.5911) (4.2423, -1.6261) (4.1208, -1.7002) (4.0735, -1.7331) knots 0 0 0 1 2 2 2
  line L160 (4.0735, -1.7331) -> (4.0529, -1.7331)
  line L161 (4.0529, -1.7331) -> (4.0529, -1.3729)
  spline S179 degree 2 poles (4.0529, -1.3729) (4.164, -1.3132) (4.5448, -1.2165) (4.7157, -1.2165) knots 0 0 0 1 2 2 2
  spline S180 degree 2 poles (4.7157, -1.2165) (4.8886, -1.2165) (5.1459, -1.2865) (5.2508, -1.3606) knots 0 0 0 1 2 2 2
  spline S181 degree 2 poles (5.2508, -1.3606) (5.362, -1.4408) (5.4773, -1.6734) (5.4773, -1.8299) knots 0 0 0 1 2 2 2
  spline S182 degree 2 poles (5.4773, -1.8299) (5.4773, -2.0398) (5.2014, -2.3568) (5.008, -2.398) knots 0 0 0 1 2 2 2
  line L162 (5.008, -2.398) -> (5.008, -2.4227)
  spline S183 degree 2 poles (5.008, -2.4227) (5.0882, -2.4391) (5.2714, -2.5132) (5.3496, -2.5873) knots 0 0 0 1 2 2 2
  spline S184 degree 2 poles (5.3496, -2.5873) (5.4279, -2.6594) (5.5267, -2.8899) (5.5267, -3.0566) knots 0 0 0 1 2 2 2
  spline S185 degree 2 poles (5.5267, -3.0566) (5.5267, -3.2275) (5.4093, -3.5177) (5.3023, -3.6289) knots 0 0 0 1 2 2 2
  spline S186 degree 2 poles (5.3023, -3.6289) (5.1912, -3.7441) (4.8762, -3.8635) (4.6766, -3.8635) knots 0 0 0 1 2 2 2
  spline S187 degree 2 poles (4.6766, -3.8635) (4.4851, -3.8635) (4.1105, -3.7709) (3.9829, -3.7071) knots 0 0 0 1 2 2 2
  line L163 (3.9829, -3.7071) -> (3.9829, -3.3469)
  line L164 (3.9829, -3.3469) -> (4.0076, -3.3469)
  spline S188 degree 2 poles (4.0076, -3.3469) (4.1146, -3.4251) (4.4769, -3.5692) (4.656, -3.5692) knots 0 0 0 1 2 2 2
  spline S189 degree 2 poles (4.656, -3.5692) (4.761, -3.5692) (4.9709, -3.5033) (5.0409, -3.4271) knots 0 0 0 1 2 2 2
  spline S190 degree 2 poles (5.0409, -3.4271) (5.1088, -3.351) (5.1809, -3.1699) (5.1809, -3.0319) knots 0 0 0 1 2 2 2
  spline S191 degree 2 poles (5.1809, -3.0319) (5.1809, -2.894) (5.1006, -2.715) (5.0285, -2.6635) knots 0 0 0 1 2 2 2
  spline S192 degree 2 poles (5.0285, -2.6635) (4.9565, -2.612) (4.761, -2.5729) (4.6457, -2.5729) knots 0 0 0 1 2 2 2
  line L165 (4.6457, -2.5729) -> (4.5016, -2.5729)
  line L166 (4.5016, -2.5729) -> (4.5016, -2.2909)
  line L167 (4.5016, -2.2909) -> (4.6148, -2.2909)
  spline S193 degree 2 poles (4.6148, -2.2909) (4.8433, -2.2909) (5.1315, -2.0728) (5.1315, -1.8649) knots 0 0 0 1 2 2 2
  spline S194 degree 2 poles (5.1315, -1.8649) (5.1315, -1.7681) (5.0574, -1.6302) (4.9977, -1.589) knots 0 0 0 1 2 2 2
  spline S195 degree 2 poles (4.9977, -1.589) (4.9339, -1.5458) (4.7774, -1.5108) (4.6889, -1.5108) knots 0 0 0 1 2 2 2
  line L168 (6.455, -3.81) -> (6.0474, -3.81)
  line L169 (6.0474, -3.81) -> (6.0474, -3.3242)
  line L170 (6.0474, -3.3242) -> (6.455, -3.3242)
  line L171 (6.455, -3.3242) -> (6.455, -3.81)
  spline S196 degree 2 poles (8.5483, -2.54) (8.5483, -3.2234) (8.1511, -3.8635) (7.7373, -3.8635) knots 0 0 0 1 2 2 2
  spline S197 degree 2 poles (7.7373, -3.8635) (7.3174, -3.8635) (6.9243, -3.211) (6.9243, -2.5421) knots 0 0 0 1 2 2 2
  spline S198 degree 2 poles (6.9243, -2.5421) (6.9243, -1.8546) (7.3215, -1.2185) (7.7373, -1.2185) knots 0 0 0 1 2 2 2
  spline S199 degree 2 poles (7.7373, -1.2185) (8.1552, -1.2185) (8.5483, -1.8772) (8.5483, -2.54) knots 0 0 0 1 2 2 2
  spline S200 degree 2 poles (8.1119, -3.3139) (8.1613, -3.1884) (8.2025, -2.8014) (8.2025, -2.54) knots 0 0 0 1 2 2 2
  spline S201 degree 2 poles (8.2025, -2.54) (8.2025, -2.2786) (8.1613, -1.8937) (8.1099, -1.764) knots 0 0 0 1 2 2 2
  spline S202 degree 2 poles (8.1099, -1.764) (8.0584, -1.6343) (7.8794, -1.5005) (7.7373, -1.5005) knots 0 0 0 1 2 2 2
  spline S203 degree 2 poles (7.7373, -1.5005) (7.5953, -1.5005) (7.4121, -1.6343) (7.3586, -1.7681) knots 0 0 0 1 2 2 2
  spline S204 degree 2 poles (7.3586, -1.7681) (7.3071, -1.8978) (7.2701, -2.293) (7.2701, -2.5421) knots 0 0 0 1 2 2 2
  spline S205 degree 2 poles (7.2701, -2.5421) (7.2701, -2.8096) (7.303, -3.1678) (7.3565, -3.3078) knots 0 0 0 1 2 2 2
  spline S206 degree 2 poles (7.3565, -3.3078) (7.4059, -3.4395) (7.5891, -3.5815) (7.7373, -3.5815) knots 0 0 0 1 2 2 2
  spline S207 degree 2 poles (7.7373, -3.5815) (7.8773, -3.5815) (8.0605, -3.4477) (8.1119, -3.3139) knots 0 0 0 1 2 2 2
  line L172 (12.1731, -3.81) -> (12.1731, -2.7067)
  spline S208 degree 2 poles (12.1731, -2.7067) (12.1731, -2.575) (12.1525, -2.3506) (12.1195, -2.2889) knots 0 0 0 1 2 2 2
  spline S209 degree 2 poles (12.1195, -2.2889) (12.0866, -2.221) (11.9611, -2.1551) (11.852, -2.1551) knots 0 0 0 1 2 2 2
  spline S210 degree 2 poles (11.852, -2.1551) (11.7532, -2.1551) (11.5267, -2.2765) (11.4074, -2.3918) knots 0 0 0 1 2 2 2
  spline S211 degree 2 poles (11.4074, -2.3918) (11.4094, -2.4206) (11.4135, -2.5009) (11.4135, -2.5544) knots 0 0 0 1 2 2 2
  line L173 (11.4135, -2.5544) -> (11.4135, -3.81)
  line L174 (11.4135, -3.81) -> (11.0924, -3.81)
  line L175 (11.0924, -3.81) -> (11.0924, -2.7067)
  spline S212 degree 2 poles (11.0924, -2.7067) (11.0924, -2.575) (11.0718, -2.3506) (11.0389, -2.2889) knots 0 0 0 1 2 2 2
  spline S213 degree 2 poles (11.0389, -2.2889) (11.006, -2.221) (10.8804, -2.1551) (10.7713, -2.1551) knots 0 0 0 1 2 2 2
  spline S214 degree 2 poles (10.7713, -2.1551) (10.6684, -2.1551) (10.4399, -2.2848) (10.3329, -2.3856) knots 0 0 0 1 2 2 2
  line L176 (10.3329, -2.3856) -> (10.3329, -3.81)
  line L177 (10.3329, -3.81) -> (10.0118, -3.81)
  line L178 (10.0118, -3.81) -> (10.0118, -1.904)
  line L179 (10.0118, -1.904) -> (10.3329, -1.904)
  line L180 (10.3329, -1.904) -> (10.3329, -2.1139)
  spline S215 degree 2 poles (10.3329, -2.1139) (10.4585, -1.9884) (10.7055, -1.8505) (10.8537, -1.8505) knots 0 0 0 1 2 2 2
  spline S216 degree 2 poles (10.8537, -1.8505) (11.0224, -1.8505) (11.2839, -2.0048) (11.3518, -2.1798) knots 0 0 0 1 2 2 2
  spline S217 degree 2 poles (11.3518, -2.1798) (11.4979, -2.0172) (11.7737, -1.8505) (11.9343, -1.8505) knots 0 0 0 1 2 2 2
  spline S218 degree 2 poles (11.9343, -1.8505) (12.0578, -1.8505) (12.2595, -1.9266) (12.3336, -2.0131) knots 0 0 0 1 2 2 2
  spline S219 degree 2 poles (12.3336, -2.0131) (12.4098, -2.0995) (12.4942, -2.3589) (12.4942, -2.5544) knots 0 0 0 1 2 2 2
  line L181 (12.4942, -2.5544) -> (12.4942, -3.81)
  line L182 (12.4942, -3.81) -> (12.1731, -3.81)
  line L183 (15.1062, -3.81) -> (15.1062, -2.7067)
  spline S220 degree 2 poles (15.1062, -2.7067) (15.1062, -2.575) (15.0856, -2.3506) (15.0527, -2.2889) knots 0 0 0 1 2 2 2
  spline S221 degree 2 poles (15.0527, -2.2889) (15.0198, -2.221) (14.8942, -2.1551) (14.7851, -2.1551) knots 0 0 0 1 2 2 2
  spline S222 degree 2 poles (14.7851, -2.1551) (14.6863, -2.1551) (14.4599, -2.2765) (14.3405, -2.3918) knots 0 0 0 1 2 2 2
  spline S223 degree 2 poles (14.3405, -2.3918) (14.3426, -2.4206) (14.3467, -2.5009) (14.3467, -2.5544) knots 0 0 0 1 2 2 2
  line L184 (14.3467, -2.5544) -> (14.3467, -3.81)
  line L185 (14.3467, -3.81) -> (14.0256, -3.81)
  line L186 (14.0256, -3.81) -> (14.0256, -2.7067)
  spline S224 degree 2 poles (14.0256, -2.7067) (14.0256, -2.575) (14.005, -2.3506) (13.9721, -2.2889) knots 0 0 0 1 2 2 2
  spline S225 degree 2 poles (13.9721, -2.2889) (13.9391, -2.221) (13.8136, -2.1551) (13.7045, -2.1551) knots 0 0 0 1 2 2 2
  spline S226 degree 2 poles (13.7045, -2.1551) (13.6016, -2.1551) (13.3731, -2.2848) (13.266, -2.3856) knots 0 0 0 1 2 2 2
  line L187 (13.266, -2.3856) -> (13.266, -3.81)
  line L188 (13.266, -3.81) -> (12.9449, -3.81)
  line L189 (12.9449, -3.81) -> (12.9449, -1.904)
  line L190 (12.9449, -1.904) -> (13.266, -1.904)
  line L191 (13.266, -1.904) -> (13.266, -2.1139)
  spline S227 degree 2 poles (13.266, -2.1139) (13.3916, -1.9884) (13.6386, -1.8505) (13.7868, -1.8505) knots 0 0 0 1 2 2 2
  spline S228 degree 2 poles (13.7868, -1.8505) (13.9556, -1.8505) (14.217, -2.0048) (14.2849, -2.1798) knots 0 0 0 1 2 2 2
  spline S229 degree 2 poles (14.2849, -2.1798) (14.4311, -2.0172) (14.7069, -1.8505) (14.8674, -1.8505) knots 0 0 0 1 2 2 2
  spline S230 degree 2 poles (14.8674, -1.8505) (14.9909, -1.8505) (15.1927, -1.9266) (15.2668, -2.0131) knots 0 0 0 1 2 2 2
  spline S231 degree 2 poles (15.2668, -2.0131) (15.3429, -2.0995) (15.4273, -2.3589) (15.4273, -2.5544) knots 0 0 0 1 2 2 2
  line L192 (15.4273, -2.5544) -> (15.4273, -3.81)
  line L193 (15.4273, -3.81) -> (15.1062, -3.81)
  line L194 (-4.162, -16.8665) -> (-5.7284, -16.8665)
  line L195 (-5.7284, -16.8665) -> (-5.7284, -16.5063)
  spline S232 degree 2 poles (-5.7284, -16.5063) (-5.5596, -16.3478) (-5.2591, -16.0535) (-5.115, -15.895) knots 0 0 0 1 2 2 2
  spline S233 degree 2 poles (-5.115, -15.895) (-4.8248, -15.5759) (-4.6128, -15.1931) (-4.6128, -14.9893) knots 0 0 0 1 2 2 2
  spline S234 degree 2 poles (-4.6128, -14.9893) (-4.6128, -14.8823) (-4.6786, -14.7217) (-4.7383, -14.6703) knots 0 0 0 1 2 2 2
  spline S235 degree 2 poles (-4.7383, -14.6703) (-4.798, -14.6188) (-4.9544, -14.5673) (-5.0491, -14.5673) knots 0 0 0 1 2 2 2
  spline S236 degree 2 poles (-5.0491, -14.5673) (-5.1397, -14.5673) (-5.3249, -14.6126) (-5.4093, -14.6476) knots 0 0 0 1 2 2 2
  spline S237 degree 2 poles (-5.4093, -14.6476) (-5.4814, -14.6764) (-5.6152, -14.7588) (-5.6563, -14.7876) knots 0 0 0 1 2 2 2
  line L196 (-5.6563, -14.7876) -> (-5.6749, -14.7876)
  line L197 (-5.6749, -14.7876) -> (-5.6749, -14.4253)
  spline S238 degree 2 poles (-5.6749, -14.4253) (-5.5699, -14.3739) (-5.1932, -14.273) (-5.0244, -14.273) knots 0 0 0 1 2 2 2
  spline S239 degree 2 poles (-5.0244, -14.273) (-4.6683, -14.273) (-4.267, -14.6497) (-4.267, -14.9708) knots 0 0 0 1 2 2 2
  spline S240 degree 2 poles (-4.267, -14.9708) (-4.267, -15.121) (-4.3369, -15.3722) (-4.3987, -15.4792) knots 0 0 0 1 2 2 2
  spline S241 degree 2 poles (-4.3987, -15.4792) (-4.4604, -15.5903) (-4.6395, -15.8085) (-4.7383, -15.9135) knots 0 0 0 1 2 2 2
  spline S242 degree 2 poles (-4.7383, -15.9135) (-4.8989, -16.0885) (-5.292, -16.4631) (-5.4093, -16.5722) knots 0 0 0 1 2 2 2
  line L198 (-5.4093, -16.5722) -> (-4.162, -16.5722)
  line L199 (-4.162, -16.5722) -> (-4.162, -16.8665)
  line L200 (-3.2769, -16.8665) -> (-3.6844, -16.8665)
  line L201 (-3.6844, -16.8665) -> (-3.6844, -16.3808)
  line L202 (-3.6844, -16.3808) -> (-3.2769, -16.3808)
  line L203 (-3.2769, -16.3808) -> (-3.2769, -16.8665)
  spline S243 degree 2 poles (-1.2247, -16.0597) (-1.2247, -16.2428) (-1.342, -16.5557) (-1.4491, -16.671) knots 0 0 0 1 2 2 2
  spline S244 degree 2 poles (-1.4491, -16.671) (-1.5561, -16.7862) (-1.8752, -16.92) (-2.0728, -16.92) knots 0 0 0 1 2 2 2
  spline S245 degree 2 poles (-2.0728, -16.92) (-2.2539, -16.92) (-2.6079, -16.8398) (-2.7376, -16.776) knots 0 0 0 1 2 2 2
  line L204 (-2.7376, -16.776) -> (-2.7376, -16.4157)
  line L205 (-2.7376, -16.4157) -> (-2.7129, -16.4157)
  spline S246 degree 2 poles (-2.7129, -16.4157) (-2.6738, -16.4446) (-2.5277, -16.5187) (-2.4391, -16.5516) knots 0 0 0 1 2 2 2
  spline S247 degree 2 poles (-2.4391, -16.5516) (-2.3383, -16.5866) (-2.1716, -16.6257) (-2.0666, -16.6257) knots 0 0 0 1 2 2 2
  spline S248 degree 2 poles (-2.0666, -16.6257) (-1.9637, -16.6257) (-1.7702, -16.5516) (-1.7002, -16.4713) knots 0 0 0 1 2 2 2
  spline S249 degree 2 poles (-1.7002, -16.4713) (-1.6364, -16.3952) (-1.5705, -16.1934) (-1.5705, -16.0576) knots 0 0 0 1 2 2 2
  spline S250 degree 2 poles (-1.5705, -16.0576) (-1.5705, -15.9217) (-1.6446, -15.7488) (-1.7146, -15.6912) knots 0 0 0 1 2 2 2
  spline S251 degree 2 poles (-1.7146, -15.6912) (-1.7866, -15.6274) (-2.0007, -15.5739) (-2.1304, -15.5739) knots 0 0 0 1 2 2 2
  spline S252 degree 2 poles (-2.1304, -15.5739) (-2.2704, -15.5739) (-2.5482, -15.6171) (-2.6326, -15.6356) knots 0 0 0 1 2 2 2
  line L206 (-2.6326, -15.6356) -> (-2.6326, -14.3265)
  line L207 (-2.6326, -14.3265) -> (-1.2391, -14.3265)
  line L208 (-1.2391, -14.3265) -> (-1.2391, -14.625)
  line L209 (-1.2391, -14.625) -> (-2.3053, -14.625)
  line L210 (-2.3053, -14.625) -> (-2.3053, -15.3022)
  spline S253 degree 2 poles (-2.3053, -15.3022) (-2.2436, -15.2939) (-2.1242, -15.2878) (-2.0748, -15.2878) knots 0 0 0 1 2 2 2
  spline S254 degree 2 poles (-2.0748, -15.2878) (-1.8793, -15.2878) (-1.6096, -15.3516) (-1.4861, -15.4463) knots 0 0 0 1 2 2 2
  spline S255 degree 2 poles (-1.4861, -15.4463) (-1.3606, -15.5409) (-1.2247, -15.8291) (-1.2247, -16.0597) knots 0 0 0 1 2 2 2
  line L211 (2.4412, -16.8665) -> (2.4412, -15.7632)
  spline S256 degree 2 poles (2.4412, -15.7632) (2.4412, -15.6315) (2.4206, -15.4072) (2.3877, -15.3454) knots 0 0 0 1 2 2 2
  spline S257 degree 2 poles (2.3877, -15.3454) (2.3547, -15.2775) (2.2292, -15.2116) (2.1201, -15.2116) knots 0 0 0 1 2 2 2
  spline S258 degree 2 poles (2.1201, -15.2116) (2.0213, -15.2116) (1.7949, -15.3331) (1.6755, -15.4483) knots 0 0 0 1 2 2 2
  spline S259 degree 2 poles (1.6755, -15.4483) (1.6776, -15.4771) (1.6817, -15.5574) (1.6817, -15.6109) knots 0 0 0 1 2 2 2
  line L212 (1.6817, -15.6109) -> (1.6817, -16.8665)
  line L213 (1.6817, -16.8665) -> (1.3606, -16.8665)
  line L214 (1.3606, -16.8665) -> (1.3606, -15.7632)
  spline S260 degree 2 poles (1.3606, -15.7632) (1.3606, -15.6315) (1.34, -15.4072) (1.307, -15.3454) knots 0 0 0 1 2 2 2
  spline S261 degree 2 poles (1.307, -15.3454) (1.2741, -15.2775) (1.1486, -15.2116) (1.0395, -15.2116) knots 0 0 0 1 2 2 2
  spline S262 degree 2 poles (1.0395, -15.2116) (0.9365, -15.2116) (0.7081, -15.3413) (0.601, -15.4421) knots 0 0 0 1 2 2 2
  line L215 (0.601, -15.4421) -> (0.601, -16.8665)
  line L216 (0.601, -16.8665) -> (0.2799, -16.8665)
  line L217 (0.2799, -16.8665) -> (0.2799, -14.9605)
  line L218 (0.2799, -14.9605) -> (0.601, -14.9605)
  line L219 (0.601, -14.9605) -> (0.601, -15.1704)
  spline S263 degree 2 poles (0.601, -15.1704) (0.7266, -15.0449) (0.9736, -14.907) (1.1218, -14.907) knots 0 0 0 1 2 2 2
  spline S264 degree 2 poles (1.1218, -14.907) (1.2906, -14.907) (1.552, -15.0614) (1.6199, -15.2363) knots 0 0 0 1 2 2 2
  spline S265 degree 2 poles (1.6199, -15.2363) (1.7661, -15.0737) (2.0419, -14.907) (2.2024, -14.907) knots 0 0 0 1 2 2 2
  spline S266 degree 2 poles (2.2024, -14.907) (2.3259, -14.907) (2.5276, -14.9831) (2.6018, -15.0696) knots 0 0 0 1 2 2 2
  spline S267 degree 2 poles (2.6018, -15.0696) (2.6779, -15.156) (2.7623, -15.4154) (2.7623, -15.6109) knots 0 0 0 1 2 2 2
  line L220 (2.7623, -15.6109) -> (2.7623, -16.8665)
  line L221 (2.7623, -16.8665) -> (2.4412, -16.8665)
  line L222 (5.3743, -16.8665) -> (5.3743, -15.7632)
  spline S268 degree 2 poles (5.3743, -15.7632) (5.3743, -15.6315) (5.3538, -15.4072) (5.3208, -15.3454) knots 0 0 0 1 2 2 2
  spline S269 degree 2 poles (5.3208, -15.3454) (5.2879, -15.2775) (5.1623, -15.2116) (5.0532, -15.2116) knots 0 0 0 1 2 2 2
  spline S270 degree 2 poles (5.0532, -15.2116) (4.9544, -15.2116) (4.728, -15.3331) (4.6086, -15.4483) knots 0 0 0 1 2 2 2
  spline S271 degree 2 poles (4.6086, -15.4483) (4.6107, -15.4771) (4.6148, -15.5574) (4.6148, -15.6109) knots 0 0 0 1 2 2 2
  line L223 (4.6148, -15.6109) -> (4.6148, -16.8665)
  line L224 (4.6148, -16.8665) -> (4.2937, -16.8665)
  line L225 (4.2937, -16.8665) -> (4.2937, -15.7632)
  spline S272 degree 2 poles (4.2937, -15.7632) (4.2937, -15.6315) (4.2731, -15.4072) (4.2402, -15.3454) knots 0 0 0 1 2 2 2
  spline S273 degree 2 poles (4.2402, -15.3454) (4.2073, -15.2775) (4.0817, -15.2116) (3.9726, -15.2116) knots 0 0 0 1 2 2 2
  spline S274 degree 2 poles (3.9726, -15.2116) (3.8697, -15.2116) (3.6412, -15.3413) (3.5342, -15.4421) knots 0 0 0 1 2 2 2
  line L226 (3.5342, -15.4421) -> (3.5342, -16.8665)
  line L227 (3.5342, -16.8665) -> (3.2131, -16.8665)
  line L228 (3.2131, -16.8665) -> (3.2131, -14.9605)
  line L229 (3.2131, -14.9605) -> (3.5342, -14.9605)